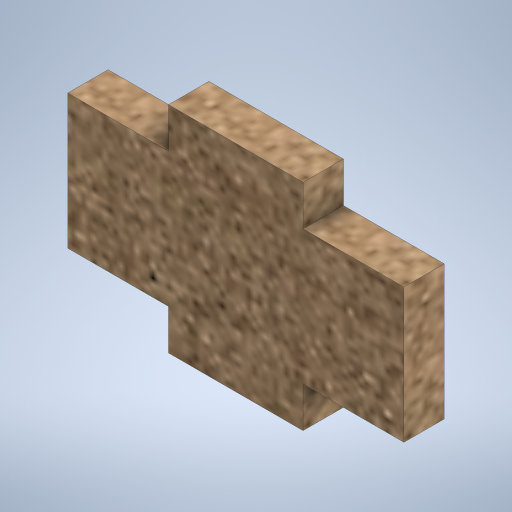
# Autodesk Inventor part: Case_Support
Saved by Autodesk Inventor 2024 (Build 280153000, 153)
## iProperties
Created: 2023-11-23
Part Number: Case_Support
Material: MDF Tablero de fibras de densidad media
Document SubType Name: Modeling
Designer: marco
Density: 0.8 g/cm^3
Appearance: Cartón - Ondulado
Author: marco
Autodesk Inventor part; units mm, degrees
ref_plane "YZ Plane" through (0, 0, 0) normal (1, 0, 0) x (0, 1, 0)
ref_plane "XZ Plane" through (0, 0, 0) normal (0, 1, 0) x (-1, 0, 0)
ref_plane "XY Plane" through (0, 0, 0) normal (0, 0, 1) x (1, 0, 0)
sketch "Boceto1" plane through (0, 0, 0) normal (0, 0, 1) x (1, 0, 0)
  line L0 (-12.5, -5) -> (-12.5, 5)
  line L1 (-5, -5) -> (-12.5, -5)
  line L2 (-5, -8) -> (-5, -5)
  line L3 (5, -8) -> (-5, -8)
  line L4 (5, -5) -> (5, -8)
  line L5 (12.5, -5) -> (5, -5)
  line L6 (12.5, 5) -> (12.5, -5)
  line L7 (5, 5) -> (12.5, 5)
  line L8 (5, 8) -> (5, 5)
  line L9 (-5, 8) -> (5, 8)
  line L10 (-5, 5) -> (-5, 8)
  line L11 (-12.5, 5) -> (-5, 5)
  point P0 (0, 0)
  point P1 (12.5, -5)
  point P2 (5, 8)
  constraints: 24 end point
extrude "Extrusión1" add sketch "Boceto1" along normal blind 3
